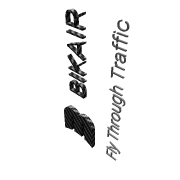
# Autodesk Inventor part: Bikair_Logo
Saved by Autodesk Inventor 2016 (Build 200138000, 138)
## iProperties
Created: 2015-05-14
Part Number: Bikair_Logo
Material: Generic
Document SubType Name: Modeling
Designer: Yann
Density: 1 g/cm^3
Appearance: Carbon Fiber
Author: Yann
Autodesk Inventor part; units mm, degrees
ref_plane "YZ Plane" through (0, 0, 0) normal (1, 0, 0) x (0, 1, 0)
ref_plane "XZ Plane" through (0, 0, 0) normal (0, 1, 0) x (-1, 0, 0)
ref_plane "XY Plane" through (0, 0, 0) normal (0, 0, 1) x (1, 0, 0)
sketch "Sketch1" plane through (0, 0, 0) normal (0, 0, 1) x (1, 0, 0)
  line L0 (0, 24.8103) -> (0, -128.2631) construction
  line L1 (-69.1744, 0) -> (69.1744, 0) construction
  circle A0 centre (0, -56.9852) radius 49.4103 construction
  line L2 (-8.7, -8.3468) -> (-8.7, -0.8651)
  line L3 (-4.5, -7.7802) -> (-4.5, -1.144)
  line L4 (-3, -7.666) -> (-3, -1.144)
  line L5 (4.5, -7.7802) -> (4.5, 2.4506)
  line L6 (8.7, -8.3468) -> (8.7, -0.711)
  line L7 (3, -7.666) -> (3, 2.4116)
  line L8 (-3, -1.144) -> (-4.5, -1.144) construction
  arc A1 (-3, -1.144) -> (-4.5, -1.144) centre (-3.75, -1.144) ccw
  arc A2 (-4.5, -7.7802) -> (-8.7, -8.3468) centre (0, -56.9852) ccw
  arc A3 (3, -7.666) -> (-3, -7.666) centre (0, -56.9852) ccw
  arc A4 (8.7, -8.3468) -> (4.5, -7.7802) centre (0, -56.9852) ccw
  arc A5 (-0.184, 1.1203) -> (-7.943, 0.7018) centre (-3.7683, -4.5606) ccw
  arc A6 (8.7, 0) -> (0, 1) centre (3.9019, -3.3989) ccw construction
  arc A7 (-7.943, 0.7018) -> (-8.7, -0.8651) centre (-6.7, -0.8651) ccw
  arc A8 (3, 2.4116) -> (0.1667, 1.1424) centre (3.9019, -3.3989) ccw
  arc A9 (8.1423, 0.6746) -> (4.5, 2.4506) centre (3.9019, -3.3989) ccw
  arc A10 (8.7, -0.711) -> (8.1423, 0.6746) centre (6.7, -0.711) ccw
  arc A11 (-0.184, 1.1203) -> (0.1667, 1.1424) centre (-0.0239, 1.3741) ccw
  point P0 (-8.7, 0)
  point P1 (8.7, 0)
  dimension "d0" = 4.2
  dimension "d1" = 1.5
  dimension "d2" = 3
  dimension "d3" = 2
  dimension "d5" = 1
  dimension "d6" = 2
  dimension "d7" = 0.3
  constraints: 35 point on circle, 14 end point, 12 centre point, 7 point on line, 7 tangent, 3 coincident, 3 perpendicular, 3 vertical, 2 concentric, 1 horizontal, 1 midpoint, 3 other
  measures "d0" distance between parallel lines of L3 L2
  measures "d1" distance between parallel lines of L3 L4
  measures "d2" distance between parallel lines of L4 L0
  measures "d3" radius of A7
  measures "d5" distance from line of A6.end L1
  measures "d6" radius of A10
  measures "d7" radius of A11
extrude "Extrusion1" [suppressed]
sketch "Sketch2" plane through (0, 0, 0) normal (0, 0, 1) x (1, 0, 0)
  line L0 (-18.7622, 0) -> (25.7675, 0) construction
  arc A0 (0, -9) -> (-11, -11.7554) centre (0, -32.3345) ccw construction
  line L1 (-11, -11.7554) -> (-11, 0)
  line L2 (-5, -9.542) -> (-5, 0)
  line L3 (-3, -9.1937) -> (-3, 0)
  arc A1 (-3, 0) -> (-5, 0) centre (-4, 0) ccw
  arc A2 (0, 4) -> (-11, 0) centre (-4.7727, 0) ccw
  arc A3 (-5, -9.542) -> (-11, -11.7554) centre (0, -32.3345) ccw
  arc A4 (0, -9) -> (-3, -9.1937) centre (0, -32.3345) ccw
  arc A5 (11, -11.7554) -> (0, -9) centre (0, -32.3345) ccw construction
  line L4 (11, -11.7554) -> (11, 0)
  line L5 (5, -9.542) -> (5, 0)
  line L6 (3, -9.1937) -> (3, 0)
  arc A6 (5, 0) -> (3, 0) centre (4, 0) ccw
  arc A7 (11, 0) -> (0, 4) centre (4.7727, 0) ccw
  arc A8 (11, -11.7554) -> (5, -9.542) centre (0, -32.3345) ccw
  arc A9 (3, -9.1937) -> (0, -9) centre (0, -32.3345) ccw
  line L7 (5.1266, 17.9652) -> (-4.8734, 17.9652)
  line L8 (-4.8734, 17.9652) -> (-4.8734, 20.9166)
  spline S0 degree 2 poles (-4.8734, 20.9166) (-4.8734, 22.5241) (-3.5461, 24.1894) (-2.26, 24.1894) knots 0 0 0 1 2 2 2
  spline S1 degree 2 poles (-2.26, 24.1894) (-1.4768, 24.1894) (-0.3309, 23.3403) (-0.0836, 22.6066) knots 0 0 0 1 2 2 2
  spline S2 degree 2 poles (-0.0836, 22.6066) (0.106, 23.4804) (1.4415, 24.5439) (2.3072, 24.5439) knots 0 0 0 1 2 2 2
  spline S3 degree 2 poles (2.3072, 24.5439) (3.6345, 24.5439) (5.1266, 22.8374) (5.1266, 21.3123) knots 0 0 0 1 2 2 2
  line L9 (5.1266, 21.3123) -> (5.1266, 17.9652)
  line L10 (0.3204, 18.8143) -> (4.4094, 18.8143)
  line L11 (4.4094, 18.8143) -> (4.4094, 21.3452)
  spline S4 degree 2 poles (4.4094, 21.3452) (4.4094, 22.4335) (3.3047, 23.703) (2.3237, 23.703) knots 0 0 0 1 2 2 2
  spline S5 degree 2 poles (2.3237, 23.703) (1.4003, 23.703) (0.3204, 22.4829) (0.3204, 21.4112) knots 0 0 0 1 2 2 2
  line L12 (0.3204, 21.4112) -> (0.3204, 18.8143)
  line L13 (-0.3886, 18.8143) -> (-0.3886, 21.1144)
  spline S6 degree 2 poles (-0.3886, 21.1144) (-0.4134, 22.1779) (-1.3614, 23.3321) (-2.2765, 23.3321) knots 0 0 0 1 2 2 2
  spline S7 degree 2 poles (-2.2765, 23.3321) (-3.2411, 23.3321) (-4.1561, 22.1367) (-4.1561, 20.9166) knots 0 0 0 1 2 2 2
  line L14 (-4.1561, 20.9166) -> (-4.1561, 18.8143)
  line L15 (-4.1561, 18.8143) -> (-0.3886, 18.8143)
  line L16 (5.1266, 27.6107) -> (5.1266, 26.7698)
  line L17 (5.1266, 26.7698) -> (-4.8734, 26.7698)
  line L18 (-4.8734, 26.7698) -> (-4.8734, 27.6107)
  line L19 (-4.8734, 27.6107) -> (5.1266, 27.6107)
  line L20 (0.1637, 32.5736) -> (1.5487, 31.1721)
  line L21 (1.5487, 31.1721) -> (5.1266, 31.1721)
  line L22 (5.1266, 31.1721) -> (5.1266, 30.323)
  line L23 (5.1266, 30.323) -> (-4.8734, 30.323)
  line L24 (-4.8734, 30.323) -> (-4.8734, 31.1721)
  line L25 (-4.8734, 31.1721) -> (0.5182, 31.1721)
  line L26 (0.5182, 31.1721) -> (-4.8734, 36.2917)
  line L27 (-4.8734, 36.2917) -> (-4.8734, 37.3551)
  line L28 (-4.8734, 37.3551) -> (-0.4216, 33.1672)
  line L29 (-0.4216, 33.1672) -> (5.1266, 37.6767)
  line L30 (5.1266, 37.6767) -> (5.1266, 36.6461)
  line L31 (5.1266, 36.6461) -> (0.1637, 32.5736)
  line L32 (2.3237, 44.5934) -> (2.3237, 40.0509)
  line L33 (2.3237, 40.0509) -> (5.1266, 39.0204)
  line L34 (5.1266, 39.0204) -> (5.1266, 38.1383)
  line L35 (5.1266, 38.1383) -> (-4.8734, 41.9223)
  line L36 (-4.8734, 41.9223) -> (-4.8734, 42.722)
  line L37 (-4.8734, 42.722) -> (5.1266, 46.506)
  line L38 (5.1266, 46.506) -> (5.1266, 45.6321)
  line L39 (5.1266, 45.6321) -> (2.3237, 44.5934)
  line L40 (1.6064, 40.3147) -> (1.6064, 44.3296)
  line L41 (1.6064, 44.3296) -> (-3.8429, 42.318)
  line L42 (-3.8429, 42.318) -> (1.6064, 40.3147)
  line L43 (5.1266, 49.0039) -> (5.1266, 48.163)
  line L44 (5.1266, 48.163) -> (-4.8734, 48.163)
  line L45 (-4.8734, 48.163) -> (-4.8734, 49.0039)
  line L46 (-4.8734, 49.0039) -> (5.1266, 49.0039)
  line L47 (0.9634, 55.459) -> (0.9634, 52.5489)
  line L48 (0.9634, 52.5489) -> (5.1266, 52.5489)
  line L49 (5.1266, 52.5489) -> (5.1266, 51.6997)
  line L50 (5.1266, 51.6997) -> (-4.8734, 51.6997)
  line L51 (-4.8734, 51.6997) -> (-4.8734, 54.9479)
  spline S8 degree 2 poles (-4.8734, 54.9479) (-4.8734, 56.5472) (-3.3235, 58.3444) (-1.9303, 58.3444) knots 0 0 0 1 2 2 2
  spline S9 degree 2 poles (-1.9303, 58.3444) (-0.9657, 58.3444) (0.5017, 57.2232) (0.782, 56.2752) knots 0 0 0 1 2 2 2
  line L52 (0.782, 56.2752) -> (5.0359, 58.7731)
  line L53 (5.0359, 58.7731) -> (5.1266, 58.7731)
  line L54 (5.1266, 58.7731) -> (5.1266, 57.8745)
  line L55 (5.1266, 57.8745) -> (0.9634, 55.459)
  line L56 (0.2462, 52.5489) -> (0.2462, 55.1375)
  spline S10 degree 2 poles (0.2462, 55.1375) (0.2462, 56.201) (-0.9657, 57.4953) (-1.9303, 57.4953) knots 0 0 0 1 2 2 2
  spline S11 degree 2 poles (-1.9303, 57.4953) (-2.9855, 57.4953) (-4.1561, 56.1515) (-4.1561, 54.9314) knots 0 0 0 1 2 2 2
  line L57 (-4.1561, 54.9314) -> (-4.1561, 52.5489)
  line L58 (-4.1561, 52.5489) -> (0.2462, 52.5489)
  point P0 (0, 0)
  point P1 (-4.8734, 16.7039)
  dimension "d10" = 4
  dimension "d11" = 9
  dimension "d13" = 2
  dimension "d17" = 6
  constraints: 24 point on circle, 12 end point, 10 centre point, 4 coincident, 3 tangent, 3 vertical, 2 point on line, 1 other
  measures "d10" distance of A2.start point (0, 0)
  measures "d11" distance of A0.start point (0, 0)
  measures "d13" distance between parallel lines of L3 L2
  measures "d17" distance between parallel lines of L1 L2
extrude "Extrusion2" add sketch "Sketch2" along normal blind 2.0625
sketch "Sketch3" plane through (0, 0, 0) normal (0, 0, 1) x (1, 0, 0)
  line L0 (23.0772, -6.8291) -> (23.0772, -9.6704)
  line L1 (23.0772, -9.6704) -> (25.9285, -9.6704)
  line L2 (25.9285, -9.6704) -> (25.9285, -10.1884)
  line L3 (25.9285, -10.1884) -> (19.8285, -10.1884)
  line L4 (19.8285, -10.1884) -> (19.8285, -6.4067)
  line L5 (19.8285, -6.4067) -> (20.266, -6.4067)
  line L6 (20.266, -6.4067) -> (20.266, -9.6704)
  line L7 (20.266, -9.6704) -> (22.6397, -9.6704)
  line L8 (22.6397, -9.6704) -> (22.6397, -6.8291)
  line L9 (22.6397, -6.8291) -> (23.0772, -6.8291)
  line L10 (25.9285, -4.9131) -> (25.9285, -5.416)
  line L11 (25.9285, -5.416) -> (19.4916, -5.416)
  line L12 (19.4916, -5.416) -> (19.4916, -4.9131)
  line L13 (19.4916, -4.9131) -> (25.9285, -4.9131)
  line L14 (25.2094, -2.117) -> (21.3975, -0.7945)
  line L15 (21.3975, -0.7945) -> (21.3975, -0.2513)
  line L16 (21.3975, -0.2513) -> (26.6979, -2.1874)
  line L17 (26.6979, -2.1874) -> (26.9343, -2.288)
  spline S0 degree 2 poles (26.9343, -2.288) (27.759, -2.6602) (27.759, -3.4396) knots 0 0 0 1 1 1
  spline S1 degree 2 poles (27.759, -3.4396) (27.759, -3.6207) (27.6987, -3.8268) knots 0 0 0 1 1 1
  line L18 (27.6987, -3.8268) -> (27.2863, -3.8319)
  line L19 (27.2863, -3.8319) -> (27.3115, -3.5704)
  spline S2 degree 2 poles (27.3115, -3.5704) (27.3115, -3.2033) (26.9494, -2.7456) (26.5018, -2.5847) knots 0 0 0 1 2 2 2
  line L20 (26.5018, -2.5847) -> (25.8933, -2.3635)
  line L21 (25.8933, -2.3635) -> (21.3975, -4.0733)
  line L22 (21.3975, -4.0733) -> (21.3975, -3.5251)
  line L23 (21.3975, -3.5251) -> (25.2094, -2.117)
  line L24 (20.266, 6.8645) -> (20.266, 4.7775)
  line L25 (20.266, 4.7775) -> (25.9285, 4.7775)
  line L26 (25.9285, 4.7775) -> (25.9285, 4.2595)
  line L27 (25.9285, 4.2595) -> (20.266, 4.2595)
  line L28 (20.266, 4.2595) -> (20.266, 2.1726)
  line L29 (20.266, 2.1726) -> (19.8285, 2.1726)
  line L30 (19.8285, 2.1726) -> (19.8285, 6.8645)
  line L31 (19.8285, 6.8645) -> (20.266, 6.8645)
  spline S3 degree 2 poles (22.1619, 8.2323) (21.7546, 8.4788) (21.312, 9.2482) (21.312, 9.7058) knots 0 0 0 1 2 2 2
  spline S4 degree 2 poles (21.312, 9.7058) (21.312, 10.435) (22.1317, 11.1491) (22.9565, 11.1541) knots 0 0 0 1 2 2 2
  line L32 (22.9565, 11.1541) -> (25.9285, 11.1541)
  line L33 (25.9285, 11.1541) -> (25.9285, 10.6512)
  line L34 (25.9285, 10.6512) -> (22.9515, 10.6512)
  spline S5 degree 2 poles (22.9515, 10.6512) (22.343, 10.6512) (21.7496, 10.1433) (21.7496, 9.5851) knots 0 0 0 1 2 2 2
  spline S6 degree 2 poles (21.7496, 9.5851) (21.7496, 9.1224) (22.3329, 8.4033) (22.8257, 8.2323) knots 0 0 0 1 2 2 2
  line L35 (22.8257, 8.2323) -> (25.9285, 8.2323)
  line L36 (25.9285, 8.2323) -> (25.9285, 7.7345)
  line L37 (25.9285, 7.7345) -> (19.4916, 7.7345)
  line L38 (19.4916, 7.7345) -> (19.4916, 8.2323)
  line L39 (19.4916, 8.2323) -> (22.1619, 8.2323)
  spline S7 degree 2 poles (21.825, 14.5335) (21.7948, 14.3776) (21.7948, 14.1966) knots 0 0 0 1 1 1
  spline S8 degree 2 poles (21.7948, 14.1966) (21.7948, 13.7289) (22.3178, 13.0802) (22.8157, 12.9393) knots 0 0 0 1 2 2 2
  line L40 (22.8157, 12.9393) -> (25.9285, 12.9393)
  line L41 (25.9285, 12.9393) -> (25.9285, 12.4415)
  line L42 (25.9285, 12.4415) -> (21.3975, 12.4415)
  line L43 (21.3975, 12.4415) -> (21.3975, 12.9293)
  line L44 (21.3975, 12.9293) -> (22.1167, 12.9393)
  spline S9 degree 2 poles (22.1167, 12.9393) (21.312, 13.3366) (21.312, 14.2167) knots 0 0 0 1 1 1
  spline S10 degree 2 poles (21.312, 14.2167) (21.312, 14.4279) (21.3674, 14.5486) knots 0 0 0 1 1 1
  line L45 (21.3674, 14.5486) -> (21.825, 14.5335)
  spline S11 degree 2 poles (23.5951, 15.0515) (22.9414, 15.0515) (21.8954, 15.5594) (21.312, 16.4847) (21.312, 17.068) knots 0 0 0 1 2 3 3 3
  spline S12 degree 2 poles (21.312, 17.068) (21.312, 17.9732) (22.5793, 19.0947) (23.6303, 19.0947) knots 0 0 0 1 2 2 2
  line L46 (23.6303, 19.0947) -> (23.736, 19.0947)
  spline S13 degree 2 poles (23.736, 19.0947) (24.3897, 19.0947) (25.4458, 18.5918) (26.014, 17.6665) (26.014, 17.0781) knots 0 0 0 1 2 3 3 3
  spline S14 degree 2 poles (26.014, 17.0781) (26.014, 16.1779) (24.7417, 15.0515) (23.6957, 15.0515) knots 0 0 0 1 2 2 2
  line L47 (23.6957, 15.0515) -> (23.5951, 15.0515)
  spline S15 degree 2 poles (23.736, 15.5544) (24.5456, 15.5544) (25.5916, 16.3942) (25.5916, 17.0781) knots 0 0 0 1 2 2 2
  spline S16 degree 2 poles (25.5916, 17.0781) (25.5916, 17.757) (24.5456, 18.5968) (23.6907, 18.5968) knots 0 0 0 1 2 2 2
  line L48 (23.6907, 18.5968) -> (23.5951, 18.5968)
  spline S17 degree 2 poles (23.5951, 18.5968) (23.0772, 18.5968) (22.2122, 18.2146) (21.7395, 17.5156) (21.7395, 17.068) knots 0 0 0 1 2 3 3 3
  spline S18 degree 2 poles (21.7395, 17.068) (21.7395, 16.3992) (22.7905, 15.5544) (23.6404, 15.5544) knots 0 0 0 1 2 2 2
  line L49 (23.6404, 15.5544) -> (23.736, 15.5544)
  spline S19 degree 2 poles (25.3552, 23.0473) (26.014, 22.5948) (26.014, 21.599) knots 0 0 0 1 1 1
  spline S20 degree 2 poles (26.014, 21.599) (26.014, 20.8749) (25.1742, 20.1206) (24.3444, 20.1155) knots 0 0 0 1 2 2 2
  line L50 (24.3444, 20.1155) -> (21.3975, 20.1155)
  line L51 (21.3975, 20.1155) -> (21.3975, 20.6134)
  line L52 (21.3975, 20.6134) -> (24.2841, 20.6134)
  spline S21 degree 2 poles (24.2841, 20.6134) (25.5765, 20.6134) (25.5765, 21.6594) knots 0 0 0 1 1 1
  spline S22 degree 2 poles (25.5765, 21.6594) (25.5765, 22.7506) (24.6763, 23.0373) knots 0 0 0 1 1 1
  line L53 (24.6763, 23.0373) -> (21.3975, 23.0373)
  line L54 (21.3975, 23.0373) -> (21.3975, 23.5402)
  line L55 (21.3975, 23.5402) -> (25.9285, 23.5402)
  line L56 (25.9285, 23.5402) -> (25.9285, 23.0524)
  line L57 (25.9285, 23.0524) -> (25.3552, 23.0473)
  spline S23 degree 2 poles (23.6203, 24.6415) (22.5542, 24.6415) (21.312, 25.5819) (21.312, 26.3915) knots 0 0 0 1 2 2 2
  spline S24 degree 2 poles (21.312, 26.3915) (21.312, 27.3168) (22.0513, 27.7996) knots 0 0 0 1 1 1
  line L58 (22.0513, 27.7996) -> (21.3975, 27.8248)
  line L59 (21.3975, 27.8248) -> (21.3975, 28.2924)
  line L60 (21.3975, 28.2924) -> (25.838, 28.2924)
  spline S25 degree 2 poles (25.838, 28.2924) (26.713, 28.2924) (27.7339, 27.3118) (27.7339, 26.477) knots 0 0 0 1 2 2 2
  spline S26 degree 2 poles (27.7339, 26.477) (27.7339, 26.0043) (27.3115, 25.1444) (26.9594, 24.898) knots 0 0 0 1 2 2 2
  line L61 (26.9594, 24.898) -> (26.6577, 25.1746)
  spline S27 degree 2 poles (26.6577, 25.1746) (27.3115, 25.7076) (27.3115, 26.4418) knots 0 0 0 1 1 1
  spline S28 degree 2 poles (27.3115, 26.4418) (27.3115, 27.0704) (26.5722, 27.7745) (25.9134, 27.7845) knots 0 0 0 1 2 2 2
  line L62 (25.9134, 27.7845) -> (25.3452, 27.7845)
  spline S29 degree 2 poles (25.3452, 27.7845) (26.014, 27.3068) (26.014, 26.3815) knots 0 0 0 1 1 1
  spline S30 degree 2 poles (26.014, 26.3815) (26.014, 25.597) (24.7568, 24.6415) (23.6857, 24.6415) knots 0 0 0 1 2 2 2
  line L63 (23.6857, 24.6415) -> (23.6203, 24.6415)
  spline S31 degree 2 poles (23.7108, 25.1494) (24.5758, 25.1494) (25.5765, 25.8434) (25.5765, 26.477) knots 0 0 0 1 2 2 2
  spline S32 degree 2 poles (25.5765, 26.477) (25.5765, 27.4023) (24.7468, 27.7845) knots 0 0 0 1 1 1
  line L64 (24.7468, 27.7845) -> (22.6397, 27.7845)
  spline S33 degree 2 poles (22.6397, 27.7845) (22.2072, 27.6085) (21.7496, 26.9497) (21.7496, 26.4821) knots 0 0 0 1 2 2 2
  spline S34 degree 2 poles (21.7496, 26.4821) (21.7496, 25.8534) (22.7402, 25.1494) (23.7108, 25.1494) knots 0 0 0 1 2 2 2
  spline S35 degree 2 poles (22.1619, 30.0978) (21.7546, 30.3442) (21.312, 31.1136) (21.312, 31.5713) knots 0 0 0 1 2 2 2
  spline S36 degree 2 poles (21.312, 31.5713) (21.312, 32.3004) (22.1317, 33.0145) (22.9565, 33.0196) knots 0 0 0 1 2 2 2
  line L65 (22.9565, 33.0196) -> (25.9285, 33.0196)
  line L66 (25.9285, 33.0196) -> (25.9285, 32.5167)
  line L67 (25.9285, 32.5167) -> (22.9515, 32.5167)
  spline S37 degree 2 poles (22.9515, 32.5167) (22.343, 32.5167) (21.7496, 32.0088) (21.7496, 31.4506) knots 0 0 0 1 2 2 2
  spline S38 degree 2 poles (21.7496, 31.4506) (21.7496, 30.9879) (22.3329, 30.2688) (22.8257, 30.0978) knots 0 0 0 1 2 2 2
  line L68 (22.8257, 30.0978) -> (25.9285, 30.0978)
  line L69 (25.9285, 30.0978) -> (25.9285, 29.5999)
  line L70 (25.9285, 29.5999) -> (19.4916, 29.5999)
  line L71 (19.4916, 29.5999) -> (19.4916, 30.0978)
  line L72 (19.4916, 30.0978) -> (22.1619, 30.0978)
  line L73 (20.266, 40.6483) -> (20.266, 38.5614)
  line L74 (20.266, 38.5614) -> (25.9285, 38.5614)
  line L75 (25.9285, 38.5614) -> (25.9285, 38.0434)
  line L76 (25.9285, 38.0434) -> (20.266, 38.0434)
  line L77 (20.266, 38.0434) -> (20.266, 35.9564)
  line L78 (20.266, 35.9564) -> (19.8285, 35.9564)
  line L79 (19.8285, 35.9564) -> (19.8285, 40.6483)
  line L80 (19.8285, 40.6483) -> (20.266, 40.6483)
  spline S39 degree 2 poles (21.825, 43.6103) (21.7948, 43.4544) (21.7948, 43.2734) knots 0 0 0 1 1 1
  spline S40 degree 2 poles (21.7948, 43.2734) (21.7948, 42.8057) (22.3178, 42.157) (22.8157, 42.0162) knots 0 0 0 1 2 2 2
  line L81 (22.8157, 42.0162) -> (25.9285, 42.0162)
  line L82 (25.9285, 42.0162) -> (25.9285, 41.5183)
  line L83 (25.9285, 41.5183) -> (21.3975, 41.5183)
  line L84 (21.3975, 41.5183) -> (21.3975, 42.0061)
  line L85 (21.3975, 42.0061) -> (22.1167, 42.0162)
  spline S41 degree 2 poles (22.1167, 42.0162) (21.312, 42.4135) (21.312, 43.2935) knots 0 0 0 1 1 1
  spline S42 degree 2 poles (21.312, 43.2935) (21.312, 43.5047) (21.3674, 43.6254) knots 0 0 0 1 1 1
  line L86 (21.3674, 43.6254) -> (21.825, 43.6103)
  spline S43 degree 2 poles (25.9285, 47.2663) (25.7173, 47.1909) (25.2949, 47.1708) knots 0 0 0 1 1 1
  spline S44 degree 2 poles (25.2949, 47.1708) (25.6419, 46.9042) (26.014, 46.0896) (26.014, 45.6319) knots 0 0 0 1 2 2 2
  spline S45 degree 2 poles (26.014, 45.6319) (26.014, 44.9782) (25.2848, 44.1685) (24.7266, 44.1685) knots 0 0 0 1 2 2 2
  spline S46 degree 2 poles (24.7266, 44.1685) (24.0628, 44.1685) (23.2934, 45.2699) (23.2934, 46.2555) knots 0 0 0 1 2 2 2
  line L87 (23.2934, 46.2555) -> (23.2934, 47.1657)
  line L88 (23.2934, 47.1657) -> (22.7754, 47.1657)
  spline S47 degree 2 poles (22.7754, 47.1657) (22.2927, 47.1657) (21.7345, 46.5673) (21.7345, 45.994) knots 0 0 0 1 2 2 2
  spline S48 degree 2 poles (21.7345, 45.994) (21.7345, 45.471) (22.2726, 44.7821) (22.6497, 44.7821) knots 0 0 0 1 2 2 2
  line L89 (22.6497, 44.7821) -> (22.6447, 44.2792)
  spline S49 degree 2 poles (22.6447, 44.2792) (22.1016, 44.2792) (21.312, 45.2849) (21.312, 46.0192) knots 0 0 0 1 2 2 2
  spline S50 degree 2 poles (21.312, 46.0192) (21.312, 46.7785) (22.0714, 47.6535) (22.7503, 47.6636) knots 0 0 0 1 2 2 2
  line L90 (22.7503, 47.6636) -> (24.8926, 47.6636)
  spline S51 degree 2 poles (24.8926, 47.6636) (25.5514, 47.6636) (25.8782, 47.8044) knots 0 0 0 1 1 1
  line L91 (25.8782, 47.8044) -> (25.9285, 47.8044)
  line L92 (25.9285, 47.8044) -> (25.9285, 47.2663)
  spline S52 degree 2 poles (25.5715, 45.6923) (25.5715, 46.1952) (25.0837, 46.9847) (24.6763, 47.1657) knots 0 0 0 1 2 2 2
  line L93 (24.6763, 47.1657) -> (23.6806, 47.1657)
  line L94 (23.6806, 47.1657) -> (23.6806, 46.2706)
  spline S53 degree 2 poles (23.6806, 46.2706) (23.6907, 45.5213) (24.2238, 44.6714) (24.6864, 44.6714) knots 0 0 0 1 2 2 2
  spline S54 degree 2 poles (24.6864, 44.6714) (25.0686, 44.6714) (25.5715, 45.2397) (25.5715, 45.6923) knots 0 0 0 1 2 2 2
  line L95 (25.9285, 49.3633) -> (21.8099, 49.3633)
  line L96 (21.8099, 49.3633) -> (21.8099, 48.614)
  line L97 (21.8099, 48.614) -> (21.3975, 48.614)
  line L98 (21.3975, 48.614) -> (21.3975, 49.3633)
  line L99 (21.3975, 49.3633) -> (20.8494, 49.3633)
  spline S55 degree 2 poles (20.8494, 49.3633) (20.1504, 49.3633) (19.4061, 50.0674) (19.4061, 50.701) knots 0 0 0 1 2 2 2
  spline S56 degree 2 poles (19.4061, 50.701) (19.4061, 50.9877) (19.4765, 51.2341) knots 0 0 0 1 1 1
  line L100 (19.4765, 51.2341) -> (19.8939, 51.1989)
  spline S57 degree 2 poles (19.8939, 51.1989) (19.8436, 50.9877) (19.8436, 50.7412) knots 0 0 0 1 1 1
  spline S58 degree 2 poles (19.8436, 50.7412) (19.8436, 50.3239) (20.3616, 49.8662) (20.8343, 49.8662) knots 0 0 0 1 2 2 2
  line L101 (20.8343, 49.8662) -> (21.3975, 49.8662)
  line L102 (21.3975, 49.8662) -> (21.3975, 50.9474)
  line L103 (21.3975, 50.9474) -> (21.8099, 50.9474)
  line L104 (21.8099, 50.9474) -> (21.8099, 49.8662)
  line L105 (21.8099, 49.8662) -> (25.9285, 49.8662)
  line L106 (25.9285, 49.8662) -> (25.9285, 49.3633)
  line L107 (25.9285, 52.2046) -> (21.8099, 52.2046)
  line L108 (21.8099, 52.2046) -> (21.8099, 51.4553)
  line L109 (21.8099, 51.4553) -> (21.3975, 51.4553)
  line L110 (21.3975, 51.4553) -> (21.3975, 52.2046)
  line L111 (21.3975, 52.2046) -> (20.8494, 52.2046)
  spline S59 degree 2 poles (20.8494, 52.2046) (20.1504, 52.2046) (19.4061, 52.9087) (19.4061, 53.5423) knots 0 0 0 1 2 2 2
  spline S60 degree 2 poles (19.4061, 53.5423) (19.4061, 53.829) (19.4765, 54.0754) knots 0 0 0 1 1 1
  line L112 (19.4765, 54.0754) -> (19.8939, 54.0402)
  spline S61 degree 2 poles (19.8939, 54.0402) (19.8436, 53.829) (19.8436, 53.5825) knots 0 0 0 1 1 1
  spline S62 degree 2 poles (19.8436, 53.5825) (19.8436, 53.1652) (20.3616, 52.7075) (20.8343, 52.7075) knots 0 0 0 1 2 2 2
  line L113 (20.8343, 52.7075) -> (21.3975, 52.7075)
  line L114 (21.3975, 52.7075) -> (21.3975, 53.7887)
  line L115 (21.3975, 53.7887) -> (21.8099, 53.7887)
  line L116 (21.8099, 53.7887) -> (21.8099, 52.7075)
  line L117 (21.8099, 52.7075) -> (25.9285, 52.7075)
  line L118 (25.9285, 52.7075) -> (25.9285, 52.2046)
  line L119 (25.9285, 55.2421) -> (25.9285, 54.7392)
  line L120 (25.9285, 54.7392) -> (21.3975, 54.7392)
  line L121 (21.3975, 54.7392) -> (21.3975, 55.2421)
  line L122 (21.3975, 55.2421) -> (25.9285, 55.2421)
  spline S63 degree 2 poles (20.085, 54.6537) (19.9442, 54.6537) (19.7481, 54.8398) (19.7481, 55.1566) (19.9442, 55.3426) (20.2308, 55.3426) (20.4219, 55.1566) (20.4219, 54.8398) (20.2308, 54.6537) (20.085, 54.6537) knots 0 0 0 1 2 3 4 5 6 7 8 8 8
  spline S64 degree 2 poles (25.5916, 58.2795) (25.5916, 58.8025) (24.9982, 59.5116) (24.5305, 59.5417) knots 0 0 0 1 2 2 2
  line L123 (24.5305, 59.5417) -> (24.5305, 60.0245)
  spline S65 degree 2 poles (24.5305, 60.0245) (24.9429, 60.0044) (25.6268, 59.5267) (26.014, 58.7321) (26.014, 58.2795) knots 0 0 0 1 2 3 3 3
  spline S66 degree 2 poles (26.014, 58.2795) (26.014, 57.3894) (24.7719, 56.3434) (23.7259, 56.3434) knots 0 0 0 1 2 2 2
  line L124 (23.7259, 56.3434) -> (23.575, 56.3434)
  spline S67 degree 2 poles (23.575, 56.3434) (22.9062, 56.3434) (21.8753, 56.8161) (21.312, 57.6911) (21.312, 58.2745) knots 0 0 0 1 2 3 3 3
  spline S68 degree 2 poles (21.312, 58.2745) (21.312, 59.0238) (22.2022, 59.9893) (22.9263, 60.0245) knots 0 0 0 1 2 2 2
  line L125 (22.9263, 60.0245) -> (22.9263, 59.5417)
  spline S69 degree 2 poles (22.9263, 59.5417) (22.3932, 59.5065) (21.7395, 58.8075) (21.7395, 58.2745) knots 0 0 0 1 2 2 2
  spline S70 degree 2 poles (21.7395, 58.2745) (21.7395, 57.5956) (22.7201, 56.8463) (23.6052, 56.8463) knots 0 0 0 1 2 2 2
  line L126 (23.6052, 56.8463) -> (23.751, 56.8463)
  spline S71 degree 2 poles (23.751, 56.8463) (24.621, 56.8463) (25.5916, 57.5956) (25.5916, 58.2795) knots 0 0 0 1 2 2 2
  point P0 (0, 0)
  point P1 (19.4061, -10.9578)
  constraints: 1 other
extrude "Extrusion3" add sketch "Sketch3" along normal blind 0.7
equation "\"d6\" = d3"
equation "\"d17\" = 2 * d16"
equation "\"d16\" = 3"
body "Solid1"
